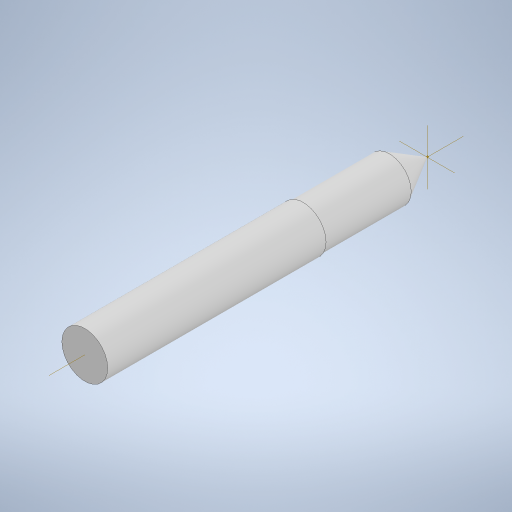
# Autodesk Inventor part: cone356
Saved by Autodesk Inventor 2023.2 (Build 272271030, 271C)
## iProperties
Created: 2023-03-03
Part Number: cone356
Material: Generisch
Document SubType Name: Modeling
Designer: mehan
Density: 1 g/cm^3
Appearance: Vorgabe
Author: mehan
Autodesk Inventor part; units mm, degrees
ref_plane "YZ Plane" through (0, 0, 0) normal (1, 0, 0) x (0, 1, 0)
ref_plane "XZ Plane" through (0, 0, 0) normal (0, 1, 0) x (-1, 0, 0)
ref_plane "XY Plane" through (0, 0, 0) normal (0, 0, 1) x (1, 0, 0)
sketch "Skizze1" plane through (0, 0, 0) normal (0, 1, 0) x (-1, 0, 0)
  line L0 (0, 0) -> (-17.8, 0) construction
  line L1 (0, 0) -> (-17.8, 30.8305)
  line L2 (0, 0) -> (35.6, 0) construction
  line L3 (-17.8, 30.8305) -> (-17.8, 101.1405)
  line L4 (-17.8, 101.1405) -> (-18.69, 101.1405)
  line L5 (0, 279.1405) -> (0, 0)
  line L6 (-18.69, 101.1405) -> (-18.69, 279.1405)
  line L7 (-18.69, 279.1405) -> (0, 279.1405)
  dimension "d0" = 17.8
  dimension "d1" = 120
  dimension "d4" = 0.89
  dimension "d6" = 178
  constraints: 16 end point, 3 horizontal, 2 perpendicular, 2 vertical, 1 equal length
  measures "d0" distance of L0.start L0.end
  measures "d1" angle of L2 L1
  measures "d4" distance of L3.end L4.end
  measures "d6" distance of L4.end L6.end
revolve "Umdrehung1" add sketch "Skizze1" angle 360 about axis through (0, 0, 279.1405) along (0, 0, -1)
